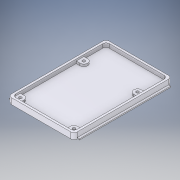
# Autodesk Inventor part: pi-holder
Saved by Autodesk Inventor 2018 (Build 220112000, 112)
## iProperties
Created: 2018-07-29
Part Number: pi-holder
Material: Generic
Document SubType Name: Modeling
Designer: jklei
Density: 1 g/cm^3
Appearance: Default
Author: jklei
Autodesk Inventor part; units mm, degrees
ref_plane "YZ Plane" through (0, 0, 0) normal (1, 0, 0) x (0, 1, 0)
ref_plane "XZ Plane" through (0, 0, 0) normal (0, 1, 0) x (-1, 0, 0)
ref_plane "XY Plane" through (0, 0, 0) normal (0, 0, 1) x (1, 0, 0)
sketch "Sketch1" plane through (0, 0, 0) normal (0, 1, 0) x (-1, 0, 0)
  line L0 (0, 0) -> (-56, 0)
  line L1 (-56, 0) -> (-56, -85.25)
  line L2 (-56, -85.25) -> (0, -85.25)
  line L3 (0, -85.25) -> (0, 0)
  dimension "d0" = 56
  dimension "d1" = 85.25
  constraints: 8 end point, 2 parallel, 1 horizontal, 1 perpendicular
  measures "d0" distance of L2.end L1.end
  measures "d1" distance of L1.end L0.end
extrude "Extrusion1" add sketch "Sketch1" along normal blind 2
sketch "Sketch2" plane through (0, 2, 0) normal (0, 1, 0) x (1, 0, 0)
  line L0 (0, 85.25) -> (0, 0) projected
  line L1 (0, 0) -> (56, 0) projected
  line L2 (56, 0) -> (56, 85.25) projected
  line L3 (56, 85.25) -> (0, 85.25) projected
  line L4 (0, 85.25) -> (0, 0) projected
  line L5 (0, 0) -> (56, 0)
  line L6 (56, 0) -> (56, 85.25)
  line L7 (56, 85.25) -> (0, 85.25)
  line L8 (0, 85.25) -> (0, 0)
  line L9 (58, -2) -> (-2, -2)
  line L10 (-2, -2) -> (-2, 87.25)
  line L11 (-2, 87.25) -> (58, 87.25)
  line L12 (58, 87.25) -> (58, -2)
  dimension "d5" = 2
  constraints: 16 end point, 2 parallel, 1 horizontal, 1 perpendicular, 3 other
  measures "d5" distance between parallel lines of L1 L9
extrude "Extrusion2" add sketch "Sketch2" along normal blind 3.5 and the other way blind 2
fillet "Fillet1" radius 3 8 edges at (-2, 2.75, 2) (58, 2.75, 2) (58, 2.75, -87.25) (-2, 2.75, -87.25) (56, 3.75, 0) (0, 3.75, 0) (56, 3.75, -85.25) (0, 3.75, -85.25)
sketch "Sketch3" plane through (0, 2, 0) normal (0, 1, 0) x (1, 0, 0)
  line L0 (1, -2) -> (55, -2) projected
  line L1 (53, 0) -> (3, 0) projected
  line L2 (0, 3) -> (0, 82.25) projected
  line L3 (-2, 84.25) -> (-2, 1) projected
  line L4 (-2, 1) -> (-2, 84.25) projected
  arc A0 (0, 3) -> (3, 0) centre (3, 3) ccw projected
  line L5 (0, 82.25) -> (0, 3) projected
  line L6 (0, 3) -> (0, 0)
  line L7 (0, 0) -> (3, 0)
  line L8 (3, 0) -> (3.5, 0)
  line L9 (3.5, 0) -> (3.5, 3.5)
  circle A1 centre (3.5, 3.5) radius 1.25
  arc A2 (53, 0) -> (56, 3) centre (53, 3) ccw projected
  line L10 (56, 3) -> (56, 0)
  line L11 (56, 0) -> (53, 0)
  line L12 (53, 0) -> (52.5, 0)
  line L13 (52.5, 0) -> (52.5, 3.5)
  circle A3 centre (52.5, 3.5) radius 1.25
  arc A4 (3, 85.25) -> (0, 82.25) centre (3, 82.25) ccw projected
  line L14 (0, 82.25) -> (0, 85.25)
  line L15 (0, 85.25) -> (3, 85.25)
  line L16 (3, 85.25) -> (53, 85.25) projected
  circle A5 centre (3.5, 61.5) radius 1.25
  line L17 (56, 82.25) -> (56, 3) projected
  line L18 (56, 82.25) -> (56, 85.25)
  line L19 (56, 85.25) -> (56.5, 85.25)
  arc A6 (56, 82.25) -> (53, 85.25) centre (53, 82.25) ccw projected
  circle A7 centre (52.5, 61.5) radius 1.25
  dimension "d9" = 0.5
  dimension "d10" = 3.5
  dimension "d11" = 2.5
  dimension "d12" = 0.5
  dimension "d13" = 3.5
  dimension "d14" = 2.5
  dimension "d17" = 2.5
  dimension "d21" = 2.5
  dimension "d24" = 61.5
  dimension "d25" = 3.5
  dimension "d26" = 61.5
  dimension "d27" = 3.5
  constraints: 24 end point, 4 centre point, 4 perpendicular, 4 point on line, 4 vertical, 3 tangent, 2 coincident, 1 point on circle
  measures "d9" distance of L7.end L8.end
  measures "d10" distance of L8.end L9.end
  measures "d11" diameter of A1
  measures "d12" distance of L1.start L12.end
  measures "d13" distance of L12.end L13.end
  measures "d14" diameter of A3
  measures "d17" diameter of A5
  measures "d21" diameter of A7
  measures "d24" distance from line of L1 A7.centre
  measures "d25" distance from line of L17 A7.centre
  measures "d26" distance from line of L1 A5.centre
  measures "d27" distance from line of L2 A5.centre
extrude "Extrusion3" cut sketch "Sketch3" against normal up to next contours A1 | A3 | A5 | A7
sketch "Sketch4" plane through (0, 2, 0) normal (0, 1, 0) x (1, 0, 0)
  circle A0 centre (3.5, 3.5) radius 1.25 projected
  arc A1 (0, 3) -> (3, 0) centre (3, 3) ccw projected
  arc A2 (7, 3.5) -> (3.5, 7) centre (3.5, 3.5) ccw
  line L0 (3, 0) -> (53, 0) projected
  line L1 (3.5, 7) -> (0, 7)
  line L2 (0, 82.25) -> (0, 3) projected
  line L3 (7, 3.5) -> (7, 0)
  circle A3 centre (3.5, 3.5) radius 1.25
  circle A4 centre (52.5, 3.5) radius 1.25 projected
  line L4 (56, 82.25) -> (56, 3) projected
  line L5 (53, 0) -> (3, 0) projected
  circle A5 centre (56.5, 3.5) radius 1.25
  circle A6 centre (3.5, 61.5) radius 1.25 projected
  circle A7 centre (52.5, 61.5) radius 1.25 projected
  arc A8 (3.5, 58) -> (3.5, 65) centre (3.5, 61.5) ccw
  arc A9 (52.5, 65) -> (52.5, 58) centre (52.5, 61.5) ccw
  line L6 (3.5, 65) -> (0, 65)
  line L7 (3.5, 58) -> (0, 58)
  line L8 (52.5, 65) -> (56, 65)
  line L9 (52.5, 58) -> (56, 58)
  circle A10 centre (3.5, 61.5) radius 1.25
  circle A11 centre (52.5, 61.5) radius 1.25
  circle A12 centre (3.5, 61.5) radius 1.25 projected
  circle A13 centre (3.5, 3.5) radius 1.25 projected
  circle A14 centre (52.5, 3.5) radius 1.25 projected
  circle A15 centre (52.5, 61.5) radius 1.25 projected
  arc A16 (3, 85.25) -> (0, 82.25) centre (3, 82.25) ccw projected
  line L10 (0, 82.25) -> (0, 3) projected
  arc A17 (0, 3) -> (3, 0) centre (3, 3) ccw projected
  line L11 (3, 0) -> (53, 0) projected
  arc A18 (53, 0) -> (56, 3) centre (53, 3) ccw projected
  line L12 (56, 3) -> (56, 82.25) projected
  arc A19 (56, 82.25) -> (53, 85.25) centre (53, 82.25) ccw projected
  line L13 (53, 85.25) -> (3, 85.25) projected
  arc A20 (53, 0) -> (56, 3) centre (53, 3) ccw projected
  arc A21 (52.5, 7) -> (49, 3.5) centre (52.5, 3.5) ccw
  line L14 (52.5, 7) -> (56, 7)
  line L15 (49, 3.5) -> (49, 0)
  point P0 (0, 0)
  dimension "d31" = 7
  dimension "d32" = 7
  dimension "d33" = 7
  constraints: 16 end point, 12 point on line, 8 centre point, 8 point on circle, 7 coincident, 4 equal radius, 3 perpendicular, 3 tangent, 2 horizontal, 1 parallel
  measures "d31" diameter of A8
  measures "d32" diameter of A9
  measures "d33" diameter of A21
extrude "Extrusion4" add sketch "Sketch4" along normal blind 2 contours L2 L1 A2 L3 L0 A1 | L2 L6 A8 L7 | L15 A21 L14 L4 A5 A18 L0 | A5 L4 A18 | L9 A9 L8 L4 picked at (55.9186, 4.05)
sketch "Sketch5" plane through (58, 0, -84.25) normal (1, 0, 0) x (0, 0, -1)
  line L0 (-83.25, 0) -> (-83.25, 5.5) projected
  line L1 (0, 0) -> (0, 5.5) projected
  line L2 (-83.25, 0) -> (0, 0)
  line L3 (0, 0) -> (0, 1)
  line L4 (0, 1) -> (-83.25, 1)
  line L5 (-83.25, 1) -> (-83.25, 0)
  point P0 (-84.25, 0)
  dimension "d36" = 1
  constraints: 8 end point, 2 parallel, 1 horizontal, 1 perpendicular, 1 point on line
  measures "d36" distance of L3.end L2.end
extrude "Extrusion5" add sketch "Sketch5" along normal blind 2
sketch "Sketch6" plane through (-2, 0, -84.25) normal (-1, 0, 0) x (0, 0, 1)
  line L0 (83.25, 1) -> (0, 1) projected
  line L1 (83.25, 0) -> (0, 0) projected
  line L2 (83.25, 5.5) -> (83.25, 0) projected
  line L3 (0, 0) -> (0, 5.5) projected
  point P0 (84.25, 0)
extrude "Extrusion6" add sketch "Sketch6" along normal blind 2
sketch "Sketch7" plane through (0, 0, 0) normal (0, -1, 0) x (1, 0, 0)
  circle A0 centre (3.5, -3.5) radius 1.25 projected
  circle A1 centre (52.5, -3.5) radius 1.25 projected
  circle A2 centre (52.5, -61.5) radius 1.25 projected
  circle A3 centre (3.5, -61.5) radius 1.25 projected
  circle A4 centre (3.5, -3.5) radius 3
  circle A5 centre (52.5, -3.5) radius 3
  circle A6 centre (52.5, -61.5) radius 3
  circle A7 centre (3.5, -61.5) radius 3
  point P0 (0, 0)
  dimension "d41" = 6
  dimension "d42" = 6
  dimension "d43" = 6
  dimension "d44" = 6
  constraints: 4 centre point, 4 coincident
  measures "d41" diameter of A4
  measures "d42" diameter of A5
  measures "d43" diameter of A6
  measures "d44" diameter of A7
extrude "Extrusion7" cut sketch "Sketch7" against normal blind 2
body "Solid1"
